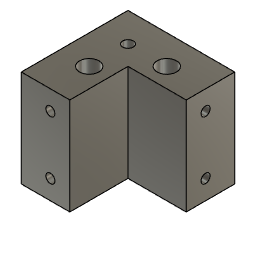
Corners_Panels_x4 (Autodesk Fusion 360 design; units mm, degrees)
Autodesk Fusion 360 part; units mm, degrees
sketch "Skizze1" plane through (0, 0, 0) normal (0, 0, 1) x (1, 0, 0)
  line L0 (0, 0) -> (20, 0)
  line L1 (20, 0) -> (20, 20)
  line L2 (20, 20) -> (0, 20)
  line L3 (0, 20) -> (0, 0)
  dimension "d1" = 20
  dimension "d2" = 20
  constraint horizontal L0
  constraint vertical L1
  constraint horizontal L2
  constraint vertical L3
  constraint coincident L0.start L3.end
  measures "d1" distance of L0.start L0.end
  measures "d2" distance of L0.start L2.end
extrude "Extrusion1" add sketch "Skizze1" along normal blind 50
extrude "Extrusion2" add 1 faces at (20, 6.6667, 16.6667) along direction (1, 0, 0) blind 20
sketch "Skizze2" plane through (0, 0, 0) normal (0, -1, 0) x (1, 0, 0)
  line L0 (0, 0) -> (40, 0)
  line L1 (40, 0) -> (40, 50)
  line L2 (40, 50) -> (0, 50)
  line L3 (0, 50) -> (0, 0)
  line L4 (0, 50) -> (20, 50)
  line L5 (20, 50) -> (20, 0)
  line L6 (20, 0) -> (0, 0)
  line L7 (0, 0) -> (0, 50)
  dimension "d7" = 20
  dimension "d8" = 50
  constraint horizontal L4
  constraint vertical L5
  constraint horizontal L6
  constraint vertical L7
  constraint coincident L2.end L3.start
  measures "d7" distance of L2.end L4.end
  measures "d8" distance of L2.end L0.start
extrude "Extrusion3" add sketch "Skizze2" along normal blind 20 contours L0 L2 L3 L4 L5 L6 L7
hole "Bohrung1" at (10, 10, 50) direction (0, 0, -1) diameter 5.5 depth 50 tip angle 118
hole "Bohrung2" at (30, 10, 50) direction (0, 0, -1) diameter 5.2 depth 50 tip angle 118 counterbore diameter 10 counterbore depth 40
hole "Bohrung3" at (10, -10, 50) direction (0, 0, -1) diameter 5.2 depth 50 tip angle 180 counterbore diameter 10 counterbore depth 40
extrude "Extrusion4" add 1 faces at (40, 6.6667, 16.6667) along direction (1, 0, 0) blind 10
extrude "Extrusion5" add 1 faces at (6.6667, -20, 16.6667) along direction (0, -1, 0) blind 10
hole "Bohrung4" at (50, 10, 40) direction (-1, 0, 0) diameter 4.7 depth 10 tip angle 180
hole "Bohrung5" at (50, 10, 10) direction (-1, 0, 0) diameter 4.7 depth 10 tip angle 180
hole "Bohrung6" at (10, -30, 40) direction (0, 1, 0) diameter 4.7 depth 10 tip angle 180
hole "Bohrung7" at (10, -30, 10) direction (0, 1, 0) diameter 4.7 depth 10 tip angle 180
extrude "Extrusion6" add 1 faces at (33.3333, 20, 33.3333) along direction (0, 1, 0) blind 5
extrude "Extrusion7" add 1 faces at (0, 6.6667, 33.3333) along direction (-1, 0, 0) blind 5
